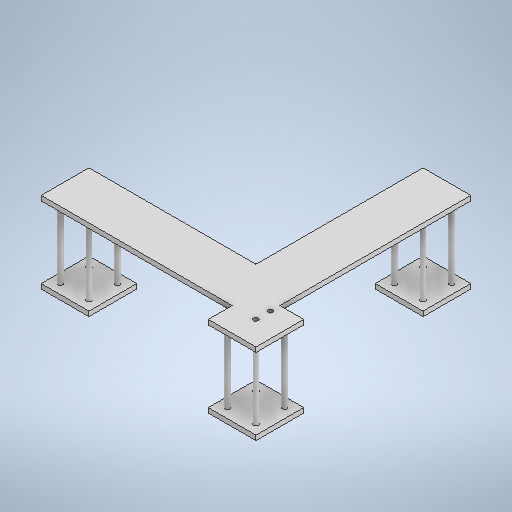
# Autodesk Inventor part: Soporte - C15
Saved by Autodesk Inventor 2025.3 (Build 293356000, 356)
## iProperties
Created: 2025-11-22
Part Number: Soporte - C15
Material: Genérico
Document SubType Name: Modeling
Designer: Gianluca Nuñez
Density: 1 g/cm^3
Appearance: Valor por defecto
Author: Gianluca Nuñez
## iProperties of the stored document Soporte - C15_3DPrint.ipt
Created: 2025-11-22
Part Number: Soporte - C15_3DPrint
Material: Genérico
Document SubType Name: Modeling
Designer: Gianluca Nuñez
Density: 1 g/cm^3
Appearance: Valor por defecto
Author: Gianluca Nuñez
Autodesk Inventor part; units mm, degrees
ref_plane "YZ Plane" through (0, 0, 0) normal (1, 0, 0) x (0, 1, 0)
ref_plane "XZ Plane" through (0, 0, 0) normal (0, 1, 0) x (-1, 0, 0)
ref_plane "XY Plane" through (0, 0, 0) normal (0, 0, 1) x (1, 0, 0)
sketch "Boceto1" plane through (0, 0, 0) normal (0, 1, 0) x (-1, 0, 0)
  line L0 (0, 0) -> (-50, 0)
  line L1 (-50, 0) -> (-50, -50)
  line L2 (-50, -50) -> (0, -50)
  line L3 (0, -50) -> (0, 0)
  dimension "d0" = 50
  dimension "d1" = 50
  constraints: 8 end point, 2 parallel, 1 horizontal, 1 perpendicular
  measures "d0" distance of L0.end L1.end
  measures "d1" distance of L1.end L2.end
extrude "Extrusión1" add sketch "Boceto1" along normal blind 5
sketch "Boceto2" plane through (0, 5, 0) normal (0, 1, 0) x (1, 0, 0)
  circle A0 centre (10, 10) radius 2.5
  line L0 (0, 50) -> (0, 0) projected
  line L1 (0, 0) -> (50, 0) projected
  circle A1 centre (10, 40) radius 2.5
  circle A2 centre (40, 10) radius 2.5
  circle A3 centre (40, 40) radius 2.5
  line L2 (50, 50) -> (0, 50) projected
  line L3 (50, 0) -> (50, 50) projected
  dimension "d4" = 5
  dimension "d5" = 10
  dimension "d6" = 10
  dimension "d7" = 5
  dimension "d8" = 5
  dimension "d9" = 5
  dimension "d10" = 10
  dimension "d11" = 10
  dimension "d12" = 10
  dimension "d13" = 10
  dimension "d14" = 10
  dimension "d15" = 10
  constraints: 4 centre point
  measures "d4" diameter of A0
  measures "d5" distance from line of L0 A0.centre
  measures "d6" distance from line of L1 A0.centre
  measures "d7" diameter of A1
  measures "d8" diameter of A2
  measures "d9" diameter of A3
  measures "d10" distance from line of L2 A1.centre
  measures "d11" distance from line of L0 A1.centre
  measures "d12" distance from line of L2 A3.centre
  measures "d13" distance from line of L3 A3.centre
  measures "d14" distance from line of L3 A2.centre
  measures "d15" distance from line of L1 A2.centre
extrude "Extrusión2" add sketch "Boceto2" along normal blind 75 contours A0 | A1 | A2 | A3
sketch "Boceto3" plane through (10, 80, -10) normal (0, 1, 0) x (1, 0, 0)
  line L0 (-10, -10) -> (40, -10) projected
  line L1 (40, 40) -> (-10, 40) projected
  line L2 (-10, -10) -> (40, -10)
  line L3 (40, -10) -> (40, 40)
  line L4 (40, 40) -> (-10, 40)
  line L5 (-10, 40) -> (-10, -10)
  constraints: 8 end point, 2 parallel, 1 horizontal, 1 perpendicular
extrude "Extrusión3" add sketch "Boceto3" along normal blind 5
sketch "Boceto4" plane through (10, 85, -10) normal (0, 1, 0) x (1, 0, 0)
  circle A0 centre (15, 15) radius 2.5
  line L0 (40, 40) -> (-10, 40) projected
  line L1 (-10, 40) -> (-10, -10) projected
  dimension "d20" = 5
  dimension "d21" = 25
  dimension "d22" = 25
  constraints: 1 centre point
  measures "d20" diameter of A0
  measures "d21" distance from line of L0 A0.centre
  measures "d22" distance from line of L1 A0.centre
extrude "Extrusión4" cut sketch "Boceto4" against normal blind 5
thread "Rosca1" size "M5x0.8" class "6H" standard "ANSI Metric M Profile" full length
sketch "Boceto7" plane through (50, 80, -50) normal (0, 0, -1) x (-1, 0, 0)
  line L0 (0, 5) -> (50, 5) projected
  line L1 (25, 5) -> (75, 5)
  line L2 (75, 5) -> (75, 0)
  line L3 (75, 0) -> (25, 0)
  line L4 (25, 0) -> (25, 5)
  point P0 (50, -80)
  dimension "d34" = 50
  dimension "d35" = 5
  constraints: 8 end point, 2 parallel, 1 horizontal, 1 midpoint, 1 perpendicular
  measures "d34" distance of L2.end L3.end
  measures "d35" distance of L1.end L2.end
extrude "Extrusión7" add sketch "Boceto7" along normal blind 200
sketch "Boceto8" plane through (0, 80, 0) normal (-1, 0, 0) x (0, 0, 1)
  line L0 (-50, 5) -> (0, 5) projected
  line L1 (-50, 0) -> (-250, 0) projected
  line L2 (-25, 5) -> (-75, 5)
  line L3 (-75, 5) -> (-75, 0)
  line L4 (-75, 0) -> (-25, 0)
  line L5 (-25, 0) -> (-25, 5)
  point P0 (0, -80)
  dimension "d38" = 50
  constraints: 8 end point, 2 parallel, 1 horizontal, 1 midpoint, 1 perpendicular, 1 point on line
  measures "d38" distance of L4.end L3.end
extrude "Extrusión8" add sketch "Boceto8" along normal blind 200
sketch "Boceto9" plane through (10, 85, -10) normal (0, 1, 0) x (1, 0, 0)
  circle A0 centre (15, 30) radius 2.5
  circle A1 centre (15, 15) radius 2.5 projected
  point P0 (-10, -10)
  dimension "d41" = 5
  dimension "d42" = 15
  dimension "d43" = 0
  constraints: 1 centre point
  measures "d41" diameter of A0
  measures "d42" distance of A1.centre A0.centre
  measures "d43" horizontal distance of A1.centre A0.centre
extrude "Extrusión9" cut sketch "Boceto9" against normal blind 10 contours A0
thread "Rosca2" size "M5x0.8" class "6H" standard "ANSI Metric M Profile" full length
sketch "Boceto10" plane through (10, 80, -10) normal (0, -1, 0) x (1, 0, 0)
  circle A0 centre (5, -230) radius 2.5
  circle A1 centre (-25, -230) radius 2.5
  circle A2 centre (-25, -200) radius 2.5
  circle A3 centre (5, -200) radius 2.5
  line L0 (15, -240) -> (-35, -240) projected
  line L1 (15, -40) -> (15, -240) projected
  line L2 (-35, -65) -> (-35, -240) projected
  line L3 (15, -40) -> (15, -240) construction
  line L4 (15, -190) -> (-35, -190) construction
  point P0 (-10, 10)
  dimension "d48" = 5
  dimension "d49" = 5
  dimension "d50" = 5
  dimension "d51" = 5
  dimension "d52" = 10
  dimension "d53" = 10
  dimension "d54" = 10
  dimension "d55" = 10
  dimension "d56" = 50
  dimension "d57" = 10
  dimension "d58" = 10
  dimension "d59" = 10
  dimension "d60" = 10
  constraints: 4 centre point, 2 end point, 2 point on line, 1 perpendicular
  measures "d48" diameter of A0
  measures "d49" diameter of A1
  measures "d50" diameter of A2
  measures "d51" diameter of A3
  measures "d52" distance from line of L0 A0.centre
  measures "d53" distance from line of L1 A0.centre
  measures "d54" distance from line of L0 A1.centre
  measures "d55" distance from line of L2 A1.centre
  measures "d56" distance between parallel lines of L0 L4
  measures "d57" distance from line of L4 A2.centre
  measures "d58" distance from line of L2 A2.centre
  measures "d59" distance from line of L4 A3.centre
  measures "d60" distance from line of L1 A3.centre
extrude "Extrusión10" add sketch "Boceto10" along normal blind 75
sketch "Boceto11" plane through (-15, 5, -240) normal (0, -1, 0) x (1, 0, 0)
  circle A0 centre (-145, 175) radius 2.5
  circle A1 centre (-175, 175) radius 2.5
  circle A2 centre (-145, 205) radius 2.5
  circle A3 centre (-175, 205) radius 2.5
  line L0 (15, 215) -> (-185, 215) projected
  line L1 (-185, 165) -> (-185, 215) projected
  line L2 (-10, 165) -> (-185, 165) construction
  line L3 (-135, 165) -> (-135, 215) construction
  point P0 (15, 240)
  dimension "d63" = 5
  dimension "d64" = 5
  dimension "d65" = 5
  dimension "d66" = 5
  dimension "d67" = 10
  dimension "d68" = 10
  dimension "d69" = 50
  dimension "d70" = 10
  dimension "d71" = 10
  dimension "d72" = 10
  dimension "d73" = 10
  dimension "d74" = 10
  dimension "d75" = 10
  constraints: 4 centre point, 2 end point, 2 point on line, 1 vertical
  measures "d63" diameter of A0
  measures "d64" diameter of A1
  measures "d65" diameter of A2
  measures "d66" diameter of A3
  measures "d67" distance from line of L0 A3.centre
  measures "d68" distance from line of L1 A3.centre
  measures "d69" distance between parallel lines of L1 L3
  measures "d70" distance from line of L0 A2.centre
  measures "d71" distance from line of L3 A2.centre
  measures "d72" distance from line of L3 A0.centre
  measures "d73" distance from line of A0.centre L2
  measures "d74" distance from line of L2 A1.centre
  measures "d75" distance from line of L1 A1.centre
extrude "Extrusión11" add sketch "Boceto11" against normal blind 75
sketch "Boceto12" plane through (-190, 5, -35) normal (0, -1, 0) x (1, 0, 0)
  line L0 (215, -15) -> (215, -215) projected
  line L1 (165, -40) -> (165, -215) projected
  line L2 (215, -215) -> (165, -215)
  line L3 (165, -215) -> (165, -165)
  line L4 (165, -165) -> (215, -165)
  line L5 (215, -165) -> (215, -215)
  line L6 (165, -40) -> (-10, -40) projected
  line L7 (190, 10) -> (-10, 10) projected
  line L8 (-10, -40) -> (40, -40)
  line L9 (40, -40) -> (40, 10)
  line L10 (40, 10) -> (-10, 10)
  line L11 (-10, 10) -> (-10, -40)
  point P0 (190, 35)
  dimension "d78" = 50
  dimension "d79" = 50
  constraints: 16 end point, 4 parallel, 2 horizontal, 2 perpendicular, 2 point on line
  measures "d78" distance of L2.end L3.end
  measures "d79" distance of L10.end L9.end
extrude "Extrusión12" add sketch "Boceto12" along normal blind 5
